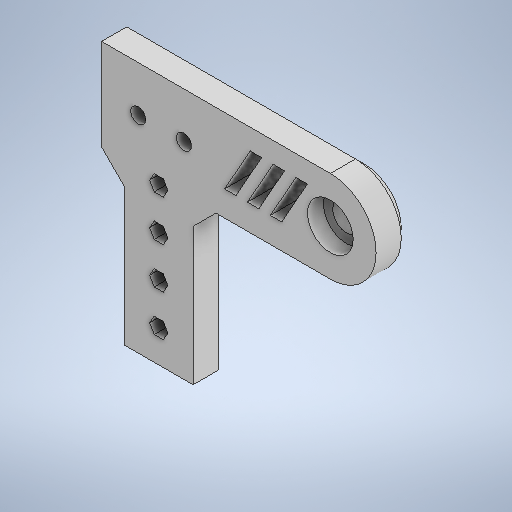
# Autodesk Inventor part: belt_leg
Saved by Autodesk Inventor 2025 (Build 290162000, 162)
## iProperties
Created: 2024-12-12
Part Number: belt_leg
Material: Všeobecné
Document SubType Name: Modeling
Designer: lukas
Density: 1 g/cm^3
Appearance: Výchozí
Author: lukas
## iProperties of the stored document belt_leg_3D tisk.ipt
Created: 2024-12-14
Part Number: belt_leg_3D tisk
Material: Všeobecné
Document SubType Name: Modeling
Designer: lukas
Density: 1 g/cm^3
Appearance: Výchozí
Author: lukas
Autodesk Inventor part; units mm, degrees
ref_plane "YZ Plane" through (0, 0, 0) normal (1, 0, 0) x (0, 1, 0)
ref_plane "XZ Plane" through (0, 0, 0) normal (0, 1, 0) x (-1, 0, 0)
ref_plane "XY Plane" through (0, 0, 0) normal (0, 0, 1) x (1, 0, 0)
sketch "Náčrt1" plane through (0, 0, 0) normal (0, 0, 1) x (1, 0, 0)
  line L0 (-74, 0) -> (94, 0) projected
  line L1 (0, 77) -> (0, -77) projected
  line L2 (-40, -55) -> (-10, -55)
  line L3 (-10, -55) -> (-10, 15)
  line L4 (-10, 15) -> (50, 15)
  line L5 (50, 15) -> (50, 55)
  line L6 (50, 55) -> (-50, 55)
  line L7 (-50, 55) -> (-50, 15)
  line L8 (-50, 15) -> (-40, 15)
  line L9 (-40, 15) -> (-40, -55)
  circle A0 centre (50, 35) radius 20
  point P0 (0, 0)
  point P1 (50, 15)
  dimension "d0" = 100
  dimension "d1" = 40
  dimension "d2" = 40
  dimension "d3" = 10
  dimension "d4" = 30
  dimension "d5" = 70
  constraints: 16 end point, 6 perpendicular, 1 horizontal, 1 midpoint, 1 vertical, 5 other
  measures "d0" distance of L5.end L6.end
  measures "d1" distance of L4.end L5.end
  measures "d2" distance of L6.end L7.end
  measures "d3" distance of L7.end L8.end
  measures "d4" distance of L2.start L2.end
  measures "d5" distance of L2.end L3.end
extrude "Vysunutí1" add sketch "Náčrt1" along normal blind 15 contours L9 L8 L7 L6 L1 L4 L3 L0 | L0 L3 L2 L9 | L1 L6 A0 L4 | A0 L5 | L5 A0
sketch "Náčrt2" plane through (0, 0, 15) normal (0, 0, 1) x (1, 0, 0)
  arc A0 (50, 15) -> (50, 55) centre (50, 35) ccw projected
  line L0 (-40, 15) -> (-40, -55) projected
  line L1 (-40, -55) -> (-10, -55) projected
  line L2 (-10, -55) -> (-10, 15) projected
  line L3 (-10, 15) -> (50, 15) projected
  arc A1 (50, 15) -> (50, 55) centre (50, 35) ccw projected
  line L4 (50, 55) -> (-50, 55) projected
  line L5 (-50, 55) -> (-50, 15) projected
  line L6 (-50, 15) -> (-40, 15) projected
  line L7 (-74, 0) -> (94, 0) projected
  line L8 (0, 77) -> (0, -77) projected
  point P0 (0, 0)
  constraints: 1 coincident
hole "Díra1" at (50, 35, 15) direction (0, 0, -1) diameter 12 end through all counterbore diameter 20 counterbore depth 7
chamfer "Zkosení1" distance 4 angle 45 8 edges at (0, 55, 0) (70, 35, 0) (20, 15, 0) (-50, 35, 0) (-40, -20, 0) (-45, 15, 0) (-10, -20, 0) (-25, -55, 0)
ref_plane "Pracovní rovina1" through (0, 0, 7.5) normal (0, 0, 1) x (1, 0, 0)
sketch "Náčrt3" plane through (0, 0, 7.5) normal (0, 0, 1) x (1, 0, 0)
  circle A0 centre (50, 35) radius 10 projected
  line L0 (-40, 15) -> (-40, -55) projected
  line L1 (-40, -55) -> (-10, -55) projected
  line L2 (-10, -55) -> (-10, 15) projected
  line L3 (-10, 15) -> (50, 15) projected
  arc A1 (50, 15) -> (50, 55) centre (50, 35) ccw projected
  line L4 (50, 55) -> (-50, 55) projected
  line L5 (-50, 55) -> (-50, 15) projected
  line L6 (-50, 15) -> (-40, 15) projected
  line L7 (0, 15) -> (-10, 5)
  line L8 (0, 15) -> (4.4525, 15) construction
  point P0 (0, 0)
  dimension "d18" = 135
  dimension "d19" = 10
  constraints: 4 end point, 2 point on line, 1 horizontal
  measures "d18" angle of L7 L8
  measures "d19" horizontal distance of L7.start L7.end
extrude "Žebro1" add sketch "Náčrt3" along normal mid plane 7 rib yes fills toward (-5.0354, 10.0354) open curves L7
sketch "Náčrt4" plane through (-10, 15, 11) normal (0, 0, 1) x (1, 0, 0)
  line L0 (0, 0) -> (10, 0) projected
  line L1 (0, -10) -> (0, 0) projected
  line L2 (10, 0) -> (0, -10) projected
  line L3 (10, 0) -> (0, 0)
  line L4 (10, 0) -> (0, -10) projected
  line L5 (0, -10) -> (10, 0)
  point P0 (10, -15)
  constraints: 4 end point, 2 collinear
extrude "Vysunutí2" add sketch "Náčrt4" along normal blind 4
sketch "Náčrt5" plane through (0, 0, 7.5) normal (0, 0, 1) x (1, 0, 0)
  circle A0 centre (50, 35) radius 10 projected
  line L0 (-40, 15) -> (-40, -55) projected
  line L1 (-40, -55) -> (-10, -55) projected
  line L2 (-10, -55) -> (-10, 5) projected
  line L3 (-10, 5) -> (0, 15) projected
  line L4 (0, 15) -> (50, 15) projected
  arc A1 (50, 15) -> (50, 55) centre (50, 35) ccw projected
  line L5 (50, 55) -> (-50, 55) projected
  line L6 (-50, 55) -> (-50, 15) projected
  line L7 (-50, 15) -> (-40, 15) projected
  line L8 (-50, 15) -> (-40, 5)
  line L9 (-50, 15) -> (-38.3899, 15) construction
  point P0 (0, 0)
  dimension "d28" = 45
  dimension "d29" = 10
  constraints: 4 end point, 2 point on line, 1 horizontal
  measures "d28" angle of L8 L9
  measures "d29" horizontal distance of L8.start L8.end
extrude "Žebro2" add sketch "Náčrt5" along normal mid plane 7 rib yes fills toward (-44.9646, 10.0354) open curves L8
sketch "Náčrt6" plane through (-50, 15, 11) normal (0, 0, 1) x (1, 0, 0)
  line L0 (10, 0) -> (10, -10) projected
  line L1 (0, 0) -> (10, 0) projected
  line L2 (10, -10) -> (0, 0) projected
  line L3 (10, 0) -> (10, -70) projected
  line L4 (0, 0) -> (10, 0)
  line L5 (10, 0) -> (10, -10)
  point P0 (50, -15)
  constraints: 4 end point, 2 point on line, 1 collinear
extrude "Vysunutí3" add sketch "Náčrt6" along normal blind 4
sketch "Náčrt8" plane through (0, 0, 0) normal (0, 0, -1) x (-1, 0, 0)
  circle A0 centre (-50, 35) radius 6 projected
  line L0 (36, 19) -> (36, -51) projected
  line L1 (46, 19) -> (36, 19) projected
  line L2 (46, 51) -> (46, 19) projected
  line L3 (-50, 51) -> (46, 51) projected
  arc A1 (-50, 51) -> (-50, 19) centre (-50, 35) ccw projected
  line L4 (14, 19) -> (-50, 19) projected
  line L5 (14, -51) -> (14, 19) projected
  line L6 (36, -51) -> (14, -51) projected
  line L7 (0, -77) -> (0, 77) projected
  line L8 (74, 0) -> (-94, 0) projected
  line L9 (-28.7327, 26) -> (-40, 46)
  line L10 (-28.7327, 26) -> (-23.7327, 26)
  line L11 (-23.7327, 26) -> (-35, 46)
  line L12 (-35, 46) -> (-40, 46)
  circle A2 centre (-50, 35) radius 6 projected
  point P0 (0, 0)
  dimension "d40" = 5
  dimension "d42" = 20
  dimension "d43" = 20
  dimension "d44" = 5
  dimension "d45" = 5
  dimension "d46" = 10
  dimension "d47" = 21.2673
  constraints: 8 end point, 1 horizontal
  measures "d40" distance of L11.end L9.end
  measures "d42" vertical distance of L9.start L9.end
  measures "d43" vertical distance of L10.end L11.end
  measures "d44" distance between parallel lines of L3 L12
  measures "d45" distance of L9.start L10.end
  measures "d46" horizontal distance of L9.end A0.centre
  measures "d47" horizontal distance of L9.start A0.centre
extrude "Vysunutí4" cut sketch "Náčrt8" against normal through all contours L9 L12 L11 L10
pattern_linear "Obdélníkové pole1" count 3 spacing 10 along (-1, 0, 0) of "Vysunutí4"
chamfer "Zkosení2" distance 1 angle 45 12 edges at (34.3663, 36, 0) (37.5, 46, 0) (29.3663, 36, 0) (26.2327, 26, 0) (24.3663, 36, 0) (27.5, 46, 0) (19.3663, 36, 0) (16.2327, 26, 0) (14.3663, 36, 0) (9.3663, 36, 0) (6.2327, 26, 0) (17.5, 46, 0)
sketch "Náčrt9" plane through (0, 0, 0) normal (0, 0, -1) x (-1, 0, 0)
  line L0 (-12.0215, 25) -> (-24.4156, 47) projected
  line L1 (-19.3171, 25) -> (-12.0215, 25) projected
  line L2 (-31.7111, 47) -> (-19.3171, 25) projected
  line L3 (-24.4156, 47) -> (-31.7111, 47) projected
  line L4 (36, 19) -> (36, -51) projected
  line L5 (46, 19) -> (36, 19) projected
  line L6 (46, 51) -> (46, 19) projected
  line L7 (-50, 51) -> (46, 51) projected
  arc A0 (-50, 51) -> (-50, 19) centre (-50, 35) ccw projected
  line L8 (14, 19) -> (-50, 19) projected
  line L9 (14, -51) -> (14, 19) projected
  line L10 (36, -51) -> (14, -51) projected
  circle A1 centre (-50, 35) radius 6 projected
  line L11 (-41.7111, 47) -> (-29.3171, 25) projected
  line L12 (-34.4156, 47) -> (-41.7111, 47) projected
  line L13 (-22.0215, 25) -> (-34.4156, 47) projected
  line L14 (-29.3171, 25) -> (-22.0215, 25) projected
  line L15 (-2.0215, 25) -> (-14.4156, 47) projected
  line L16 (-9.3171, 25) -> (-2.0215, 25) projected
  line L17 (-21.7111, 47) -> (-9.3171, 25) projected
  line L18 (-14.4156, 47) -> (-21.7111, 47) projected
  line L19 (0, -77) -> (0, 77) projected
  line L20 (74, 0) -> (-94, 0) projected
  line L21 (27, 16.4641) -> (29, 13)
  line L22 (29, 13) -> (27, 9.5359)
  line L23 (27, 9.5359) -> (23, 9.5359)
  line L24 (23, 9.5359) -> (21, 13)
  line L25 (21, 13) -> (23, 16.4641)
  line L26 (23, 16.4641) -> (27, 16.4641)
  point P0 (0, 0)
  point P1 (25, 13)
  dimension "d58" = 4
  dimension "d59" = 6
  dimension "d60" = 11
  dimension "d70" = 3.4641
  constraints: 12 end point, 13 other
  measures "d58" distance of L25.end L21.start
  measures "d59" distance from line of point (25, 13) L5
  measures "d60" distance from line of L9 point (25, 13)
  measures "d70" vertical distance of L23.end L24.end
extrude "Vysunutí5" cut sketch "Náčrt9" against normal through all contours L21 L22 L23 L24 L25 L26
chamfer "Zkosení3" distance 1 angle 45 6 edges at (-25, 16.4641, 0) (-28, 14.7321, 0) (-28, 11.2679, 0) (-25, 9.5359, 0) (-22, 11.2679, 0) (-22, 14.7321, 0)
pattern_linear "Obdélníkové pole2" count 4 spacing 18 along (0, -1, 0) of "Vysunutí5", "Zkosení3"
sketch "Náčrt10" plane through (0, 0, 0) normal (0, 0, -1) x (-1, 0, 0)
  line L0 (27.5774, -9.4641) -> (30.1547, -5) projected
  line L1 (22.4226, -9.4641) -> (27.5774, -9.4641) projected
  line L2 (19.8453, -5) -> (22.4226, -9.4641) projected
  line L3 (22.4226, -0.5359) -> (19.8453, -5) projected
  line L4 (27.5774, -0.5359) -> (22.4226, -0.5359) projected
  line L5 (30.1547, -5) -> (27.5774, -0.5359) projected
  line L6 (-2.0215, 25) -> (-14.4156, 47) projected
  line L7 (-9.3171, 25) -> (-2.0215, 25) projected
  line L8 (-21.7111, 47) -> (-9.3171, 25) projected
  line L9 (-14.4156, 47) -> (-21.7111, 47) projected
  line L10 (-41.7111, 47) -> (-29.3171, 25) projected
  line L11 (-34.4156, 47) -> (-41.7111, 47) projected
  line L12 (-22.0215, 25) -> (-34.4156, 47) projected
  line L13 (-29.3171, 25) -> (-22.0215, 25) projected
  circle A0 centre (-50, 35) radius 6 projected
  line L14 (36, 19) -> (36, -51) projected
  line L15 (46, 19) -> (36, 19) projected
  line L16 (46, 51) -> (46, 19) projected
  line L17 (-50, 51) -> (46, 51) projected
  arc A1 (-50, 51) -> (-50, 19) centre (-50, 35) ccw projected
  line L18 (14, 19) -> (-50, 19) projected
  line L19 (14, -51) -> (14, 19) projected
  line L20 (36, -51) -> (14, -51) projected
  line L21 (-12.0215, 25) -> (-24.4156, 47) projected
  line L22 (-19.3171, 25) -> (-12.0215, 25) projected
  line L23 (-31.7111, 47) -> (-19.3171, 25) projected
  line L24 (-24.4156, 47) -> (-31.7111, 47) projected
  line L25 (22.4226, 17.4641) -> (19.8453, 13) projected
  line L26 (27.5774, 17.4641) -> (22.4226, 17.4641) projected
  line L27 (30.1547, 13) -> (27.5774, 17.4641) projected
  line L28 (27.5774, 8.5359) -> (30.1547, 13) projected
  line L29 (22.4226, 8.5359) -> (27.5774, 8.5359) projected
  line L30 (19.8453, 13) -> (22.4226, 8.5359) projected
  line L31 (27.5774, -27.4641) -> (30.1547, -23) projected
  line L32 (22.4226, -27.4641) -> (27.5774, -27.4641) projected
  line L33 (19.8453, -23) -> (22.4226, -27.4641) projected
  line L34 (22.4226, -18.5359) -> (19.8453, -23) projected
  line L35 (27.5774, -18.5359) -> (22.4226, -18.5359) projected
  line L36 (30.1547, -23) -> (27.5774, -18.5359) projected
  point P0 (0, 0)
  point P1 (34, 35)
  dimension "d71" = 16
  dimension "d72" = 12
  measures "d71" distance from line of L17 point (34, 35)
  measures "d72" distance from line of L16 point (34, 35)
hole "Díra2" at (-34, 35, 0) direction (0, 0, 1) diameter 6.6 end through all counterbore diameter 12.6001 counterbore depth 6 clearance for "Strojní šroub se zápustnou hlavou" size "M6" standard "Ansi M metrický profil"
pattern_linear "Obdélníkové pole3" count 2 spacing 20 along (1, 0, 0) of "Díra2"
